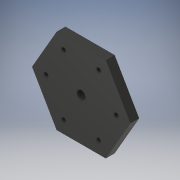
# Autodesk Inventor part: TS02
Saved by Autodesk Inventor 2017 (Build 210142000, 142)
## iProperties
Created: 2018-10-24
Part Number: TS02
Material: ABS Plastic
Document SubType Name: Modeling
Designer: Dell
Density: 1.06 g/cm^3
Appearance: Smooth - Black
Author: Dell
Autodesk Inventor part; units mm, degrees
ref_plane "YZ Plane" through (0, 0, 0) normal (1, 0, 0) x (0, 1, 0)
ref_plane "XZ Plane" through (0, 0, 0) normal (0, 1, 0) x (-1, 0, 0)
ref_plane "XY Plane" through (0, 0, 0) normal (0, 0, 1) x (1, 0, 0)
sketch "Sketch1" plane through (0, 0, 0) normal (0, 0, 1) x (1, 0, 0)
  line L0 (56, 0) -> (28, -48.4974)
  line L1 (28, -48.4974) -> (-28, -48.4974)
  line L2 (-28, -48.4974) -> (-56, 0)
  line L3 (-56, 0) -> (-28, 48.4974)
  line L4 (-28, 48.4974) -> (28, 48.4974)
  line L5 (28, 48.4974) -> (56, 0)
  circle A0 centre (0, 0) radius 10
  circle A1 centre (0, 0) radius 17.5
  circle A2 centre (0, 0) radius 30
  line L6 (0, 17.5) -> (0, 30)
  line L7 (0, -17.5) -> (0, -30)
  dimension "d0" = 112
  dimension "d1" = 20
  dimension "d2" = 35
  dimension "d3" = 60
  constraints: 16 end point, 4 coincident, 4 point on circle, 3 centre point, 2 point on line, 1 horizontal alignment, 1 vertical, 1 vertical alignment, 13 other
  measures "d0" distance of L0.start L2.end
  measures "d1" diameter of A0
  measures "d2" diameter of A1
  measures "d3" diameter of A2
extrude "Extrusion1" add sketch "Sketch1" along normal blind 10 contours L0 L1 L2 L3 L4 L5 | A1 | A1 L6 A2 L7 | A1 L7 A2 L6
extrude "Extrusion2" add sketch "Sketch1" against normal blind 10 contours A1 L6 A2 L7 picked at (25.4364, -3.5232)
sketch "Sketch2" plane through (0, 0, -10) normal (0, 0, -1) x (-1, 0, 0)
  arc A0 (0, 17.5) -> (0, -17.5) centre (0, 0) ccw projected
  line L0 (0, 17.5) -> (0, 30) projected
  arc A1 (0, 30) -> (0, -30) centre (0, 0) ccw projected
  line L1 (0, -30) -> (0, -17.5) projected
  arc A2 (-1, 28.9828) -> (-1, -28.9828) centre (0, 0) ccw
  line L2 (-1, 28.9828) -> (-1, 18.473)
  arc A3 (-1, 18.473) -> (-1, -18.473) centre (0, 0) ccw
  line L3 (-1, -18.473) -> (-1, -28.9828)
  dimension "d8" = 1
  constraints: 4 end point, 4 point on circle, 2 centre point, 3 other
  measures "d8" radial gap between concentric circles of A1 A2
extrude "Extrusion3" cut sketch "Sketch2" against normal blind 10
sketch "Sketch3" plane through (0, 0, 0) normal (0, 0, -1) x (-1, 0, 0)
  line L0 (45.7735, 0) -> (42.8868, -5)
  line L1 (42.8868, -5) -> (37.1132, -5)
  line L2 (37.1132, -5) -> (34.2265, 0)
  line L3 (34.2265, 0) -> (37.1132, 5)
  line L4 (37.1132, 5) -> (42.8868, 5)
  line L5 (42.8868, 5) -> (45.7735, 0)
  line L6 (22.8868, 39.641) -> (25.7735, 34.641)
  line L7 (25.7735, 34.641) -> (22.8868, 29.641)
  line L8 (22.8868, 29.641) -> (17.1132, 29.641)
  line L9 (17.1132, 29.641) -> (14.2265, 34.641)
  line L10 (14.2265, 34.641) -> (17.1132, 39.641)
  line L11 (17.1132, 39.641) -> (22.8868, 39.641)
  line L12 (-22.8868, 39.641) -> (-17.1132, 39.641)
  line L13 (-17.1132, 39.641) -> (-14.2265, 34.641)
  line L14 (-14.2265, 34.641) -> (-17.1132, 29.641)
  line L15 (-17.1132, 29.641) -> (-22.8868, 29.641)
  line L16 (-22.8868, 29.641) -> (-25.7735, 34.641)
  line L17 (-25.7735, 34.641) -> (-22.8868, 39.641)
  line L18 (-45.7735, 0) -> (-42.8868, 5)
  line L19 (-42.8868, 5) -> (-37.1132, 5)
  line L20 (-37.1132, 5) -> (-34.2265, 0)
  line L21 (-34.2265, 0) -> (-37.1132, -5)
  line L22 (-37.1132, -5) -> (-42.8868, -5)
  line L23 (-42.8868, -5) -> (-45.7735, 0)
  line L24 (-22.8868, -39.641) -> (-25.7735, -34.641)
  line L25 (-25.7735, -34.641) -> (-22.8868, -29.641)
  line L26 (-22.8868, -29.641) -> (-17.1132, -29.641)
  line L27 (-17.1132, -29.641) -> (-14.2265, -34.641)
  line L28 (-14.2265, -34.641) -> (-17.1132, -39.641)
  line L29 (-17.1132, -39.641) -> (-22.8868, -39.641)
  line L30 (22.8868, -39.641) -> (17.1132, -39.641)
  line L31 (17.1132, -39.641) -> (14.2265, -34.641)
  line L32 (14.2265, -34.641) -> (17.1132, -29.641)
  line L33 (17.1132, -29.641) -> (22.8868, -29.641)
  line L34 (22.8868, -29.641) -> (25.7735, -34.641)
  line L35 (25.7735, -34.641) -> (22.8868, -39.641)
  point P0 (0, 0)
  point P1 (40, 0)
  point P2 (20, 34.641)
  point P3 (-20, 34.641)
  point P4 (-40, 0)
  point P5 (-20, -34.641)
  point P6 (20, -34.641)
  dimension "d11" = 10
  dimension "d12" = 40
  dimension "d15" = 360
  constraints: 72 end point, 2 horizontal alignment, 92 other
  measures "d11" distance between parallel lines of L1 L4
  measures "d12" distance of point (0, 0) point (40, 0)
extrude "Extrusion4" cut sketch "Sketch3" against normal blind 5
sketch "Sketch4" plane through (0, 0, 0) normal (0, 0, -1) x (-1, 0, 0)
  circle A0 centre (40, 0) radius 2.5
  circle A1 centre (20, 34.641) radius 2.5
  circle A2 centre (-20, 34.641) radius 2.5
  circle A3 centre (-40, 0) radius 2.5
  circle A4 centre (-20, -34.641) radius 2.5
  circle A5 centre (20, -34.641) radius 2.5
  point P0 (0, 0)
  dimension "d19" = 5
  dimension "d20" = 40
  dimension "d23" = 360
  constraints: 6 centre point, 1 horizontal alignment, 13 other
  measures "d19" diameter of A0
  measures "d20" distance of A0.centre point (0, 0)
extrude "Extrusion5" cut sketch "Sketch4" against normal through all
sketch "Sketch5" plane through (0, 0, 10) normal (0, 0, 1) x (1, 0, 0)
  circle A0 centre (0, 0) radius 5
  circle A1 centre (0, 0) radius 10 projected
  dimension "d27" = 10
  constraints: 1 centre point, 1 coincident
  measures "d27" diameter of A0
extrude "Extrusion6" add sketch "Sketch5" against normal blind 20
sketch "Sketch6" plane through (0, 0, 0) normal (0, 1, 0) x (-1, 0, 0)
  line L0 (5, -10) -> (-5, -10)
  circle A0 centre (0, -7.5) radius 1.5
  line L1 (5, -10) -> (-5, -10) projected
  point P0 (0, 0)
  point P1 (0, -10)
  dimension "d30" = 3
  dimension "d31" = 2.5
  constraints: 2 end point, 2 midpoint, 1 centre point, 1 point on line, 1 vertical alignment
  measures "d30" diameter of A0
  measures "d31" distance from line of L0 A0.centre
extrude "Extrusion7" cut sketch "Sketch6" along normal mid plane 25
pattern_circular "Circular Pattern1" count 3 over 360 about axis through (0, 0, 10) along (0, 0, -1) of "Extrusion7"
sketch "Sketch7" plane through (0, 0, 0) normal (0, 0, -1) x (-1, 0, 0)
  arc A0 (-1, 28.9828) -> (-1, -28.9828) centre (0, 0) ccw projected
  line L0 (-29.9612, 1.5) -> (-28.9612, 1.5)
  line L1 (-28.9612, 1.5) -> (-28.9612, -1.5)
  line L2 (-28.9612, -1.5) -> (-29.9612, -1.5)
  line L3 (-29.9612, -1.5) -> (-29.9612, 1.5)
  point P0 (-28.9612, 0)
  point P1 (-29, 0)
  dimension "d37" = 1
  dimension "d38" = 3
  constraints: 8 end point, 2 parallel, 2 point on circle, 1 horizontal, 1 horizontal alignment, 1 midpoint, 1 perpendicular
  measures "d37" distance of L0.start L0.end
  measures "d38" distance of L2.end L0.start
extrude "Extrusion8" add sketch "Sketch7" along normal blind 10
sketch "Sketch8" plane through (1, -28.9828, -10) normal (-1, 0, 0) x (0, 0, 1)
  line L0 (2.5, 7.7549) -> (7.5, 7.7549)
  line L1 (7.5, 7.7549) -> (7.5, 2.7549)
  line L2 (7.5, 2.7549) -> (2.5, 2.7549)
  line L3 (2.5, 2.7549) -> (2.5, 7.7549)
  line L4 (0, 0) -> (0, 10.5098) projected
  line L5 (0, 10.5098) -> (10, 10.5098) projected
  line L6 (0, 57.9655) -> (10, 57.9655) projected
  line L7 (0, 47.4557) -> (0, 57.9655) projected
  line L8 (2.5, 55.2106) -> (7.5, 55.2106)
  line L9 (7.5, 55.2106) -> (7.5, 50.2106)
  line L10 (7.5, 50.2106) -> (2.5, 50.2106)
  line L11 (2.5, 50.2106) -> (2.5, 55.2106)
  point P0 (10, 28.9828)
  point P1 (2.5, 5.2549)
  point P2 (0, 5.2549)
  point P3 (5, 7.7549)
  point P4 (5, 10.5098)
  point P5 (5, 55.2106)
  point P6 (5, 57.9655)
  point P7 (2.5, 52.7106)
  point P8 (0, 52.7106)
  dimension "d41" = 5
  dimension "d42" = 5
  dimension "d43" = 5
  dimension "d44" = 5
  constraints: 16 end point, 8 midpoint, 4 parallel, 2 horizontal, 2 horizontal alignment, 2 perpendicular, 2 vertical alignment
  measures "d41" distance of L1.end L2.end
  measures "d42" distance of L0.end L1.end
  measures "d43" distance of L8.end L9.end
  measures "d44" distance of L8.start L8.end
extrude "Extrusion9" add sketch "Sketch8" along normal blind 0.5
fillet "Fillet1" radius 2 4 edges at (1, -28.9828, -5) (1, -18.473, -5) (1, 18.473, -5) (1, 28.9828, -5)
body "Solid1"
